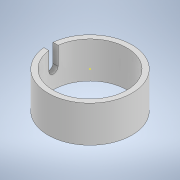
# Autodesk Inventor part: mediuminsert1
Saved by Autodesk Inventor 2022.1 (Build 261234000, 234)
## iProperties
Created: 2022-02-10
Part Number: mediuminsert1
Material: Generic
Document SubType Name: Modeling
Designer: 25lh02
Density: 1 g/cm^3
Appearance: Default
Author: 25lh02
Autodesk Inventor part; units mm, degrees
ref_plane "YZ Plane" through (0, 0, 0) normal (1, 0, 0) x (0, 1, 0)
ref_plane "XZ Plane" through (0, 0, 0) normal (0, 1, 0) x (-1, 0, 0)
ref_plane "XY Plane" through (0, 0, 0) normal (0, 0, 1) x (1, 0, 0)
sketch "Sketch1" plane through (0, 0, 0) normal (0, 1, 0) x (-1, 0, 0)
  circle A0 centre (0, 0) radius 12.827
  circle A1 centre (0, 0) radius 14.605
  dimension "d0" = 29.21
  dimension "d1" = 25.654
  constraints: 2 centre point, 2 coincident
  measures "d0" diameter of A1
  measures "d1" diameter of A0
extrude "Extrusion1" add sketch "Sketch1" along normal blind 12.7
sketch "Sketch2" plane through (0, 12.7, 0) normal (0, 1, 0) x (1, 0, 0)
  point P0 (0, 0)
sketch "Sketch3" plane through (0, 0, 0) normal (1, 0, 0) x (0, 1, 0)
  line L0 (12.7, 12.827) -> (12.7, -12.827) projected
  line L1 (12.7, 1.5875) -> (6.35, 1.5875)
  line L2 (6.35, -1.5875) -> (12.7, -1.5875)
  line L3 (12.7, 1.5875) -> (12.7, -1.5875)
  arc A0 (6.35, 1.5875) -> (6.35, -1.5875) centre (6.35, 0) ccw
  point P0 (0, 0)
  point P1 (9.525, -1.5875)
  point P2 (12.7, 0)
  dimension "d4" = 3.175
  dimension "d5" = 6.35
  constraints: 6 end point, 2 midpoint, 2 point on circle, 2 point on line, 2 tangent, 1 centre point, 1 horizontal, 1 horizontal alignment, 1 perpendicular
  measures "d4" distance from line of point (9.525, -1.587) L1
  measures "d5" distance of point (12.7, 0) A0.centre
extrude "Extrusion2" cut sketch "Sketch3" against normal blind 19.05
body "Solid1"
